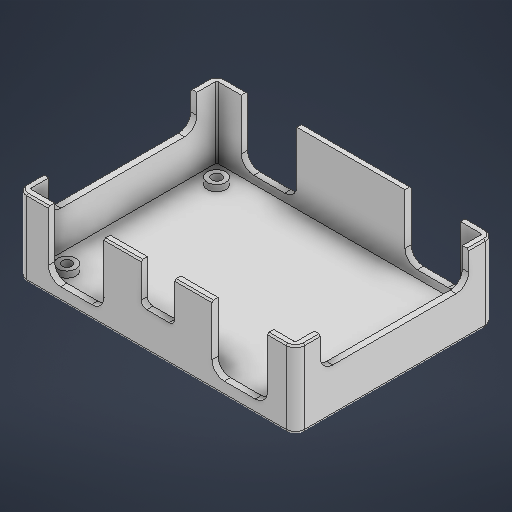
# Autodesk Inventor part: cutie
Saved by Autodesk Inventor 2026 (Build 300175000, 175)
## iProperties
Created: 2026-01-23
Part Number: cutie
Material: Generic
Document SubType Name: Modeling
Designer: neago
Density: 1 g/cm^3
Appearance: Default
Author: neago
## iProperties of the stored document cutie_3DPrint.ipt
Created: 2026-01-24
Part Number: cutie_3DPrint
Material: Generic
Document SubType Name: Modeling
Designer: neago
Density: 1 g/cm^3
Appearance: Default
Author: neago
Autodesk Inventor part; units mm, degrees
ref_plane "YZ Plane" through (0, 0, 0) normal (1, 0, 0) x (0, 1, 0)
ref_plane "XZ Plane" through (0, 0, 0) normal (0, 1, 0) x (-1, 0, 0)
ref_plane "XY Plane" through (0, 0, 0) normal (0, 0, 1) x (1, 0, 0)
sketch "Sketch1" plane through (0, 0, 0) normal (0, 1, 0) x (-1, 0, 0)
  line L0 (-42.0064, -29.8829) -> (-42.0064, 29.6171)
  line L1 (-42.0064, 29.6171) -> (42.9936, 29.6171)
  line L2 (42.9936, 29.6171) -> (42.9936, -29.8829)
  line L3 (42.9936, -29.8829) -> (-42.0064, -29.8829)
  circle A0 centre (-36.5064, 24.1171) radius 1.6
  circle A1 centre (-36.5064, -24.3829) radius 1.6
  circle A2 centre (37.4936, -24.3829) radius 1.6
  circle A3 centre (37.4936, 24.1171) radius 1.6
  line L4 (-42.5064, -29.8829) -> (-42.5064, 30.1171)
  line L5 (-42.5064, 30.1171) -> (43.4936, 30.1171)
  line L6 (43.4936, -29.8829) -> (43.4936, 30.1171)
  line L7 (-42.5064, -30.3829) -> (43.4936, -30.3829)
  line L8 (-42.5064, -29.8829) -> (-42.5064, -30.3829)
  line L9 (43.4936, -30.3829) -> (43.4936, -29.8829)
  line L10 (-44.5064, -32.3829) -> (45.4936, -32.3829)
  line L11 (45.4936, -32.3829) -> (45.4936, 32.1171)
  line L12 (45.4936, 32.1171) -> (-44.5064, 32.1171)
  line L13 (-44.5064, 32.1171) -> (-44.5064, -32.3829)
  point P0 (0, 0)
  dimension "d0" = 0.5
  dimension "d1" = 0.5
  dimension "d2" = 0.5
  dimension "d3" = 0.5
  dimension "d4" = 2
  dimension "d5" = 2
  dimension "d6" = 2
  dimension "d7" = 2
  constraints: 28 end point, 4 centre point, 3 vertical, 2 horizontal, 2 parallel, 2 perpendicular, 1 collinear
  measures "d0" distance between parallel lines of L4 L0
  measures "d1" distance between parallel lines of L5 L1
  measures "d2" distance between parallel lines of L2 L6
  measures "d3" distance between parallel lines of L3 L7
  measures "d4" distance between parallel lines of L7 L10
  measures "d5" distance between parallel lines of L13 L4
  measures "d6" distance between parallel lines of L5 L12
  measures "d7" distance between parallel lines of L6 L11
extrude "Extrusion1" add sketch "Sketch1" along normal blind 25 contours L13 L12 L11 L10
extrude "Extrusion2" add sketch "Sketch1" along normal blind 2 contours L0 L1 L2 L3 | L4 L5 L6 L9 L7 L8
fillet "Fillet1" radius 3 4 edges at (44.5064, 12.5, 32.1171) (44.5064, 12.5, -32.3829) (-45.4936, 12.5, -32.3829) (-45.4936, 12.5, 32.1171)
fillet "Fillet2" radius 1 8 edges at (43.6277, 0, 31.2384) (44.5064, 0, -0.1329) (43.6277, 0, -31.5042) (-0.4936, 0, -32.3829) (-44.615, 0, -31.5042) (-45.4936, 0, -0.1329) (-44.615, 0, 31.2384) (-0.4936, 0, 32.1171)
chamfer "Chamfer1" distance 0.5 angle 45 8 edges at (-0.4936, 25, 32.1171) (43.6277, 25, 31.2384) (44.5064, 25, -0.1329) (43.6277, 25, -31.5042) (-0.4936, 25, -32.3829) (-44.615, 25, -31.5042) (-45.4936, 25, -0.1329) (-44.615, 25, 31.2384)
fillet "Fillet3" radius 0.5 1 edges at (42.5064, 13.5, 30.1171)
fillet "Fillet4" radius 0.5 1 edges at (42.5064, 13.5, -30.3829)
fillet "Fillet5" radius 0.5 1 edges at (-43.4936, 13.5, -30.3829)
fillet "Fillet6" radius 0.5 1 edges at (-43.4936, 13.5, 30.1171)
sketch "Sketch2" plane through (0, 2, 0) normal (0, 1, 0) x (1, 0, 0)
  circle A0 centre (36.5064, -24.1171) radius 1.6 projected
  circle A1 centre (-37.4936, -24.1171) radius 1.6 projected
  circle A2 centre (-37.4936, 24.3829) radius 1.6 projected
  circle A3 centre (36.5064, 24.3829) radius 1.6 projected
  circle A4 centre (36.5064, -24.1171) radius 3
  circle A5 centre (-37.4936, -24.1171) radius 3
  circle A6 centre (-37.4936, 24.3829) radius 3
  circle A7 centre (36.5064, 24.3829) radius 3
  point P0 (0, 0)
  dimension "d21" = 6
  dimension "d22" = 6
  dimension "d23" = 6
  dimension "d24" = 6
  constraints: 4 centre point, 4 coincident
  measures "d21" diameter of A4
  measures "d22" diameter of A5
  measures "d23" diameter of A6
  measures "d24" diameter of A7
extrude "Extrusion3" add sketch "Sketch2" along normal blind 2
sketch "Sketch3" plane through (41.5064, 1, -32.3829) normal (0, 0, -1) x (-1, 0, 0)
  point P0 (41.5064, -1)
sketch "Sketch4" plane through (-45.4936, 1, -29.3829) normal (-1, 0, 0) x (0, 0, 1)
  line L0 (49.3829, 17.5) -> (9.3829, 17.5) construction
  line L1 (49.3829, 13.5) -> (9.3829, 13.5)
  line L2 (9.3829, 21.5) -> (49.3829, 21.5)
  arc A0 (49.3829, 13.5) -> (49.3829, 21.5) centre (49.3829, 17.5) ccw
  arc A1 (9.3829, 21.5) -> (9.3829, 13.5) centre (9.3829, 17.5) ccw
  line L3 (0, 23.5) -> (58.5, 23.5) projected
  line L4 (5.3829, 17.5) -> (5.3829, 24)
  line L5 (53.3829, 17.5) -> (53.3829, 24)
  line L6 (59, 24) -> (-0.5, 24) projected
  line L7 (5.3829, 24) -> (53.3829, 24)
  line L8 (61.5, 0) -> (61.5, 23.5) projected
  line L9 (29.3829, -1) -> (29.3829, 24)
  point P0 (29.3829, 17.5)
  point P1 (5.3829, 24)
  point P2 (29.3829, 11.5)
  dimension "d27" = 2
  dimension "d28" = 8
  dimension "d38" = 48
  dimension "d39" = 0
  constraints: 16 end point, 6 point on circle, 5 tangent, 3 midpoint, 3 perpendicular, 2 centre point, 1 horizontal, 1 parallel, 1 point on line, 1 vertical
  measures "d27" distance between parallel lines of L3 L2
  measures "d28" distance between parallel lines of L1 L2
  measures "d38" distance of L5.start L4.start
  measures "d39" horizontal distance of point (29.383, 11.5) point (29.383, 17.5)
extrude "Extrusion4" cut sketch "Sketch4" against normal blind 200 contours L1 L9 L2 A0 | L1 A1 L2 L9
extrude "Extrusion5" cut sketch "Sketch4" against normal blind 200 contours A0 L2 L9 L3 L5 | L2 A1 L4 L3 L9 | L3 L9 L6 L5 | L3 L4 L6 L9
sketch "Sketch5" plane through (41.5064, 1, -32.3829) normal (0, 0, -1) x (-1, 0, 0)
  line L0 (73, 7.5) -> (63, 7.5) construction
  line L1 (73, 11.5) -> (63, 11.5)
  line L2 (63, 3.5) -> (73, 3.5)
  arc A0 (73, 3.5) -> (73, 11.5) centre (73, 7.5) ccw
  arc A1 (63, 11.5) -> (63, 3.5) centre (63, 7.5) ccw
  line L3 (41.5064, -1) -> (41.5064, 23.5)
  line L4 (0, 23.5) -> (84, 23.5) projected
  line L5 (10.0127, 7.5) -> (20.0127, 7.5) construction
  line L6 (10.0127, 11.5) -> (20.0127, 11.5)
  line L7 (20.0127, 3.5) -> (10.0127, 3.5)
  arc A2 (10.0127, 11.5) -> (10.0127, 3.5) centre (10.0127, 7.5) ccw
  arc A3 (20.0127, 3.5) -> (20.0127, 11.5) centre (20.0127, 7.5) ccw
  line L8 (0, -1) -> (84, -1) projected
  line L9 (6.0127, 7.5) -> (6.0127, 24)
  line L10 (84.5, 24) -> (-0.5, 24) projected
  line L11 (24.0127, 7.5) -> (24.0127, 24)
  line L12 (6.0127, 24) -> (24.0127, 24)
  line L13 (59, 7.5) -> (59, 24)
  line L14 (77, 7.5) -> (77, 24)
  line L15 (59, 24) -> (77, 24)
  line L16 (59, 24) -> (59, 15.5271)
  line L17 (59, 15.5271) -> (77, 15.5271)
  line L18 (77, 15.5271) -> (77, 24)
  line L19 (6.0127, 24) -> (24.0127, 24)
  line L20 (59, 24) -> (77, 24)
  line L21 (68, 7.5) -> (68, 24) construction
  line L22 (15.0127, 7.5) -> (15.0127, 24) construction
  line L23 (84, 23.5) -> (84, 0) projected
  point P0 (84, 11.75)
  dimension "d40" = 5
  dimension "d41" = 8
  dimension "d42" = 4.5
  dimension "d45" = 7
  constraints: 44 end point, 12 point on circle, 7 symmetric about line, 5 parallel, 5 point on line, 5 tangent, 4 centre point, 4 midpoint, 4 perpendicular, 2 collinear, 2 vertical, 1 horizontal, 2 other
  measures "d40" distance of L21.start L0.end
  measures "d41" diameter of A1
  measures "d42" distance between parallel lines of L8 L2
  measures "d45" horizontal distance of point (84, 11.75) L14.start
extrude "Extrusion6" cut sketch "Sketch5" against normal blind 200 contours A0 L2 A1 L1 | L1 A1 L13 L17 L14 A0 | L17 L13 L4 L14 | L4 L13 L10 L14 | L11 A3 L6 A2 L9 L4 | L4 L9 L10 L11 | A3 L7 A2 L6
sketch "Sketch6" plane through (-42.4936, 1, 32.1171) normal (0, 0, 1) x (1, 0, 0)
  line L0 (46.1174, 12.771) -> (38.8698, 12.771) construction
  line L1 (46.1174, 11) -> (38.8698, 11)
  line L2 (38.8698, 14.5419) -> (46.1174, 14.5419)
  arc A0 (46.1174, 11) -> (46.1174, 14.5419) centre (46.1174, 12.771) ccw
  arc A1 (38.8698, 14.5419) -> (38.8698, 11) centre (38.8698, 12.771) ccw
  line L3 (37.0989, 12.771) -> (37.0989, 32.771)
  line L4 (37.0989, 32.771) -> (47.8884, 32.771)
  line L5 (47.8884, 32.771) -> (47.8884, 12.771)
  arc A2 (21, 3.5) -> (25, 7.5) centre (21, 7.5) ccw projected
  line L6 (84.5, 1) -> (-0.5, 1) projected
  point P0 (42.4936, -1)
  point P1 (42.4936, 12.771)
  point P2 (42.4936, 11)
  point P3 (42.4936, 14.5419)
  dimension "d46" = 3.5419
  dimension "d50" = 20
  dimension "d51" = 10
  constraints: 14 end point, 6 point on circle, 5 tangent, 3 midpoint, 2 centre point, 1 horizontal, 1 parallel, 1 perpendicular, 1 vertical
  measures "d46" distance of point (42.494, 11) point (42.494, 14.542)
  measures "d50" distance of L3.start L3.end
  measures "d51" distance between parallel lines of L6 L1
extrude "Extrusion7" cut sketch "Sketch6" against normal blind 15
body "Solid1"
